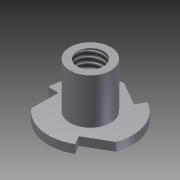
# Autodesk Inventor part: 6895_insert
Saved by Autodesk Inventor 2011 SP1 (Build 150282100, 282)
## iProperties
Created: 2013-09-15
Part Number: 6895_insert
Catalog Web Link: www.cadenas.de
Description: 6895, 6896, 6595, 6596_insert-High-Cycle Bearing Pads
Vendor: 8020
Document SubType Name: Modeling
Designer: PARTuser1
Manufacturer: 8020
Density: 1 g/cm^3
Category: PARTsolutions
Company: 8020
Title: 6895_insert
Author: Cadenas PARTsolutions
Comments: High-Cycle Bearing Pads
PSOL_IDENT_0: {$CADENAS_DATA\23d-libs\8020\inch\linear_motion\6895_insert.prj},184 {VTYP=3D},{NB=6895_insert},{LIN
PSOL_IDENT_1: A=6895_insert},{NN=6895, 6896, 6595, 6596_insert},{DATE=22.08.2012},{GEOMDATE=13.12.2011 07:18:00},{
PSOL_IDENT_2: VERSION=},{LINEID=10},{LINESUBID=-1},{WBVAR=BR,COL}  {NB=6895_insert},{LINA=6895_insert},{KT=DUMMY},
PSOL_IDENT_3: {PN=6895},{BR=1},{COL=1},{J=0.243},{L=10-32},{L1=0.190}
CNS_NT: High-Cycle Bearing Pads
CNS_NB: 6895_insert
CNS_NBSYN: $PN._insert
CNS_LINA: 6895_insert
CNS_PN: 6895
CNS_BR: No
CNS_COL: White
CNS_J: 0.243
CNS_L: 10-32
CNS_L1: 0.190
SUPPLIER: 8020
ARTICLENO: 6895_insert
BOMINFO: 6895_insert
CREATOR: CADENAS GmbH
Autodesk Inventor part; units mm, degrees
sketch "Sketch_1" plane through (0, 0, 0) normal (0, 0, 1) x (1, 0, 0)
  line L0 (0, -1.27) -> (0, 6.858)
  line L1 (0, 6.858) -> (3.0861, 6.858)
  line L2 (3.0861, 6.858) -> (3.0861, 0)
  line L3 (3.0861, 0) -> (6.35, 0)
  line L4 (6.35, 0) -> (6.35, -1.27)
  line L5 (6.35, -1.27) -> (0, -1.27)
  line L6 (0, -1.27) -> (0, 6.858)
  constraints: 14 end point
revolve "Revolution1" add sketch "Sketch_1" angle 360 about axis through (0, -1.27, 0) along (0, -1, 0)
sketch "Sketch2" plane through (0, -1.27, 0) normal (0, -1, 0) x (1, 0, 0)
  point P0 (0, 0)
hole "Drilling 1" at (0, -1.27, 0) direction (0, 1, 0) diameter 3.9624 depth 8.128 countersink diameter 4.826 countersink angle 90 thread size "10-32 UNF" class "2B" standard "ANSI Unified Screw Threads"
sketch "Sketch_3" plane through (0, 0, 0) normal (0, 1, 0) x (-1, 0, 0)
  circle A0 centre (0, 0) radius 8.89
  line L0 (6.35, 0) -> (4.826, 0)
  line L1 (4.826, 0) -> (4.826, 4.127)
  arc A1 (4.826, 4.127) -> (-3.175, 5.4993) centre (0, 0) ccw
  line L2 (-3.175, 5.4993) -> (-2.413, 4.1794)
  line L3 (-2.413, 4.1794) -> (-5.9871, 2.1159)
  arc A2 (-5.9871, 2.1159) -> (-3.175, -5.4993) centre (0, 0) ccw
  line L4 (-3.175, -5.4993) -> (-2.413, -4.1794)
  line L5 (-2.413, -4.1794) -> (1.1611, -6.2429)
  arc A3 (1.1611, -6.2429) -> (6.35, 0) centre (0, 0) ccw
  constraints: 12 end point, 6 point on circle, 4 centre point
extrude "Extrusion1" cut sketch "Sketch_3" against normal blind 2.54
ref_plane "insert_XY" through (0, 0, 0) normal (0, 1, 0) x (1, 0, 0)
ref_plane "insert_YZ" through (0, 0, 0) normal (1, 0, 0) x (0, 0, -1)
ref_plane "insert_ZX" through (0, 0, 0) normal (0, 0, -1) x (0, 1, 0)
body "Solid1"
